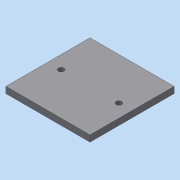
# Autodesk Inventor part: Part6
Saved by Autodesk Inventor 2016 SP1 (Build 200210100, 210)
## iProperties
Created: 2016-03-17
Part Number: Part6
Material: Generic
Document SubType Name: Modeling
Designer: Mohamed A.
Density: 1 g/cm^3
Appearance: Default
Author: Mohamed A.
Autodesk Inventor part; units mm, degrees
ref_plane "YZ Plane" through (0, 0, 0) normal (1, 0, 0) x (0, 1, 0)
ref_plane "XZ Plane" through (0, 0, 0) normal (0, 1, 0) x (-1, 0, 0)
ref_plane "XY Plane" through (0, 0, 0) normal (0, 0, 1) x (1, 0, 0)
sketch "Sketch1" plane through (0, 0, 0) normal (0, 0, 1) x (1, 0, 0)
  line L0 (7.5, 25) -> (-7.5, 25) construction
  line L1 (-7.5, 25) -> (-7.5, -25) construction
  line L2 (-7.5, -25) -> (7.5, -25) construction
  line L3 (7.5, -25) -> (7.5, 25) construction
  circle A0 centre (13.75, 3.4269) radius 1.35 projected
  circle A1 centre (-13.75, 3.4269) radius 1.35 projected
  line L4 (20, 13.4269) -> (-20, 13.4269) construction
  line L5 (-20, 13.4269) -> (-20, -6.5731) construction
  line L6 (-20, -6.5731) -> (20, -6.5731) construction
  line L7 (20, -6.5731) -> (20, 13.4269) construction
  line L8 (20, -16.5731) -> (-20, -16.5731)
  line L9 (-20, -16.5731) -> (-20, 23.4269)
  line L10 (-20, 23.4269) -> (20, 23.4269)
  line L11 (20, 23.4269) -> (20, -16.5731)
  line L12 (-20, 3.4269) -> (20, 3.4269) construction
  circle A2 centre (13.75, 18.4269) radius 1.35 projected
  circle A3 centre (-13.75, 18.4269) radius 1.35 projected
  circle A4 centre (-13.75, -11.5731) radius 1.35 projected
  circle A5 centre (13.75, -11.5731) radius 1.35 projected
  point P0 (0, 0)
  dimension "d0" = 20
  dimension "d1" = 40
  constraints: 10 end point, 4 perpendicular, 2 midpoint, 2 point on line, 1 collinear, 1 other
  measures "d0" distance between parallel lines of L6 L4
  measures "d1" distance between parallel lines of L8 L10
extrude "Extrusion1" add sketch "Sketch1" along normal blind 3
equation "\"d1\" = 2 * d0"
body "Solid1"
